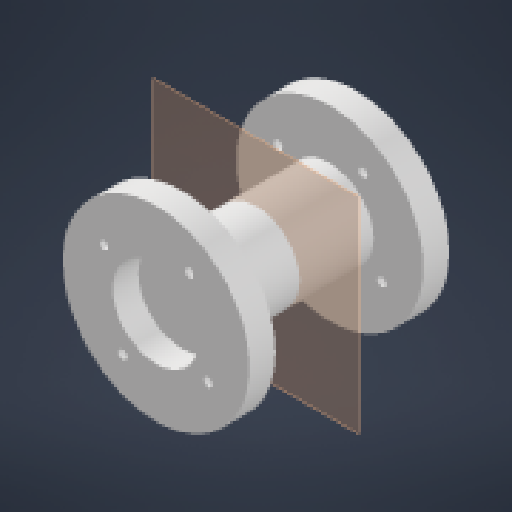
# Autodesk Inventor part: Pulley Mechanism
Saved by Autodesk Inventor 2023.6 (Build 276521000, 521)
## iProperties
Created: 2026-03-05
Part Number: Pulley Mechanism
Material: Generic
Document SubType Name: Modeling
Designer: user
Density: 1 g/cm^3
Appearance: Default
Author: user
Autodesk Inventor part; units mm, degrees
ref_plane "YZ Plane" through (0, 0, 0) normal (1, 0, 0) x (0, 1, 0)
ref_plane "XZ Plane" through (0, 0, 0) normal (0, 1, 0) x (-1, 0, 0)
ref_plane "XY Plane" through (0, 0, 0) normal (0, 0, 1) x (1, 0, 0)
sketch "Sketch1" plane through (0, 0, 0) normal (0, 0, 1) x (1, 0, 0)
  circle A0 centre (65.2764, 18.7667) radius 10.75 projected
  circle A1 centre (59.2964, 22.5941) radius 0.5 projected
  circle A2 centre (69.1038, 24.7468) radius 0.5 projected
  circle A3 centre (71.2565, 14.9393) radius 0.5 projected
  circle A4 centre (61.449, 12.7867) radius 0.5 projected
  circle A5 centre (65.2764, 18.7667) radius 7.1
  circle A6 centre (65.2764, 18.7667) radius 5
  point P0 (0, 0)
  dimension "d0" = 14.2
  dimension "d1" = 21.5
  dimension "d2" = 10
  constraints: 2 coincident, 1 centre point, 3 other
  measures "d1" diameter of A0
  measures "d2" diameter of A6
extrude "Extrusion1" add sketch "Sketch1" along normal blind 3 contours A0 | A1 A5 A2 A3 A4
sketch "Sketch2" plane through (65.2764, 18.7667, 0) normal (0, 0, -1) x (-1, 0, 0)
  circle A0 centre (0, 0) radius 5 projected
  point P0 (65.2764, -18.7667)
extrude "Extrusion2" add sketch "Sketch2" against normal blind 20
ref_plane "Work Plane1" through (65.2764, 18.7667, 11.5) normal (0, 0, 1) x (1, 0, 0)
mirror "Mirror1" about plane through (65.2764, 18.7667, 11.5) normal (0, 0, 1) of "Extrusion1"
body "Solid1"
